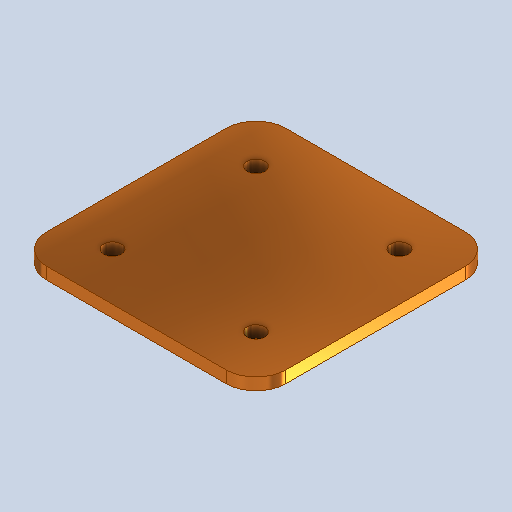
# Autodesk Inventor part: 26
Saved by Autodesk Inventor 2025.1 (Build 291241000, 241)
## iProperties
Created: 2024-09-17
Part Number: 26
Material: Gold
Document SubType Name: Modeling
Designer: ffogue
Density: 19.3 g/cm^3
Appearance: Metal 1600F Hot
Author: ffogue
Autodesk Inventor part; units mm, degrees
ref_plane "YZ Plane" through (0, 0, 0) normal (1, 0, 0) x (0, 1, 0)
ref_plane "XZ Plane" through (0, 0, 0) normal (0, 1, 0) x (-1, 0, 0)
ref_plane "XY Plane" through (0, 0, 0) normal (0, 0, 1) x (1, 0, 0)
sketch "Sketch1" plane through (0, 0, 0) normal (0, 0, 1) x (1, 0, 0)
  line L0 (-20, -20) -> (20, -20)
  line L1 (20, -20) -> (20, 20)
  line L2 (20, 20) -> (-20, 20)
  line L3 (-20, 20) -> (-20, -20)
  line L4 (-20, -20) -> (20, 20) construction
  line L5 (20, -20) -> (-20, 20) construction
  line L6 (-12, -12) -> (12, -12) construction
  line L7 (12, -12) -> (12, 12) construction
  line L8 (12, 12) -> (-12, 12) construction
  line L9 (-12, 12) -> (-12, -12) construction
  line L10 (-12, -12) -> (12, 12) construction
  line L11 (12, -12) -> (-12, 12) construction
  point P0 (0, 0)
  dimension "d0" = 40
  dimension "d1" = 40
  dimension "d2" = 24
  dimension "d3" = 24
  constraints: 24 end point, 4 coincident, 4 midpoint, 4 parallel, 2 horizontal, 2 perpendicular
  measures "d0" distance of L1.end L2.end
  measures "d1" distance of L2.end L0.start
  measures "d2" distance of L7.end L8.end
  measures "d3" distance of L8.end L6.start
extrude "Extrusion1" add sketch "Sketch1" against normal blind 2
hole "Hole1" at (-12, 12, 0) at (12, 12, 0) at (12, -12, 0) at (-12, -12, 0) direction (0, 0, -1) diameter 3 depth 2
fillet "Fillet1" radius 5 4 edges at (20, 20, -1) (20, -20, -1) (-20, -20, -1) (-20, 20, -1)
body "Solid1"
